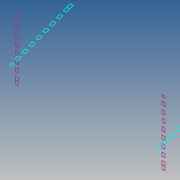
# Autodesk Inventor part: KB33-046-004-017 - Крышка наклонная
Saved by Autodesk Inventor 2020 (Build 240168000, 168)
## iProperties
Created: 2021-06-26
Part Number: KB33-046-004-017 - Крышка наклонная
Material: Типовые
Document SubType Name: Modeling
Designer: Петров Иван
Mass: 69.7839 g
Surface Area: 377.297 cm^2
Volume: 69.7839 cm^3
Density: 1 g/cm^3
Appearance: По умолчанию
Author: Петров Иван
Autodesk Inventor part; units mm, degrees
ref_plane "YZ Plane" through (0, 0, 0) normal (1, 0, 0) x (0, 1, 0)
ref_plane "XZ Plane" through (0, 0, 0) normal (0, 1, 0) x (-1, 0, 0)
ref_plane "XY Plane" through (0, 0, 0) normal (0, 0, 1) x (1, 0, 0)
sketch "Эскиз1" plane through (0, 0, 0) normal (0, 0, 1) x (1, 0, 0)
  line L0 (0, -87.7141) -> (4, -87.7141) projected
  line L1 (4, -87.7141) -> (4, -82.7141) projected
  line L2 (4, -82.7141) -> (0, -82.7141) projected
  line L3 (0, -82.7141) -> (0, -87.7141) projected
  line L4 (4, -77.7141) -> (0, -77.7141) projected
  line L5 (0, -82.7141) -> (0, -77.7141) projected
  line L6 (0, -82.7141) -> (4, -82.7141) projected
  line L7 (4, -77.7141) -> (4, -82.7141) projected
  line L8 (4, -67.7141) -> (0, -67.7141) projected
  line L9 (0, -72.7141) -> (0, -67.7141) projected
  line L10 (0, -72.7141) -> (4, -72.7141) projected
  line L11 (4, -67.7141) -> (4, -72.7141) projected
  line L12 (4, -57.7141) -> (0, -57.7141) projected
  line L13 (0, -62.7141) -> (0, -57.7141) projected
  line L14 (0, -62.7141) -> (4, -62.7141) projected
  line L15 (4, -57.7141) -> (4, -62.7141) projected
  line L16 (4, -47.7141) -> (0, -47.7141) projected
  line L17 (0, -52.7141) -> (0, -47.7141) projected
  line L18 (0, -52.7141) -> (4, -52.7141) projected
  line L19 (4, -47.7141) -> (4, -52.7141) projected
  line L20 (4, -37.7141) -> (0, -37.7141) projected
  line L21 (0, -42.7141) -> (0, -37.7141) projected
  line L22 (0, -42.7141) -> (4, -42.7141) projected
  line L23 (4, -37.7141) -> (4, -42.7141) projected
  line L24 (4, -27.7141) -> (0, -27.7141) projected
  line L25 (0, -32.7141) -> (0, -27.7141) projected
  line L26 (0, -32.7141) -> (4, -32.7141) projected
  line L27 (4, -27.7141) -> (4, -32.7141) projected
  line L28 (4, -17.7141) -> (0, -17.7141) projected
  line L29 (0, -22.7141) -> (0, -17.7141) projected
  line L30 (0, -22.7141) -> (4, -22.7141) projected
  line L31 (4, -17.7141) -> (4, -22.7141) projected
  line L32 (4, -7.7141) -> (0, -7.7141) projected
  line L33 (0, -12.7141) -> (0, -7.7141) projected
  line L34 (0, -12.7141) -> (4, -12.7141) projected
  line L35 (4, -7.7141) -> (4, -12.7141) projected
  line L36 (0, -2.7141) -> (4, -2.7141) projected
  line L37 (4, 0) -> (4, -2.7141) projected
  line L38 (0, 0) -> (4, 0) projected
  line L39 (0, -2.7141) -> (0, 0) projected
  line L40 (-199, -2.7141) -> (-195, -2.7141) projected
  line L41 (-195, 0) -> (-195, -2.7141) projected
  line L42 (-199, 0) -> (-195, 0) projected
  line L43 (-199, -2.7141) -> (-199, 0) projected
  line L44 (-195, -7.7141) -> (-199, -7.7141) projected
  line L45 (-199, -12.7141) -> (-199, -7.7141) projected
  line L46 (-199, -12.7141) -> (-195, -12.7141) projected
  line L47 (-195, -7.7141) -> (-195, -12.7141) projected
  line L48 (-195, -17.7141) -> (-199, -17.7141) projected
  line L49 (-199, -22.7141) -> (-199, -17.7141) projected
  line L50 (-199, -22.7141) -> (-195, -22.7141) projected
  line L51 (-195, -17.7141) -> (-195, -22.7141) projected
  line L52 (-195, -27.7141) -> (-199, -27.7141) projected
  line L53 (-199, -32.7141) -> (-199, -27.7141) projected
  line L54 (-199, -32.7141) -> (-195, -32.7141) projected
  line L55 (-195, -27.7141) -> (-195, -32.7141) projected
  line L56 (-195, -77.7141) -> (-199, -77.7141) projected
  line L57 (-199, -82.7141) -> (-199, -77.7141) projected
  line L58 (-199, -82.7141) -> (-195, -82.7141) projected
  line L59 (-195, -77.7141) -> (-195, -82.7141) projected
  line L60 (-195, -67.7141) -> (-199, -67.7141) projected
  line L61 (-199, -72.7141) -> (-199, -67.7141) projected
  line L62 (-199, -72.7141) -> (-195, -72.7141) projected
  line L63 (-195, -67.7141) -> (-195, -72.7141) projected
  line L64 (-195, -57.7141) -> (-199, -57.7141) projected
  line L65 (-199, -62.7141) -> (-199, -57.7141) projected
  line L66 (-199, -62.7141) -> (-195, -62.7141) projected
  line L67 (-195, -57.7141) -> (-195, -62.7141) projected
  line L68 (-199, -52.7141) -> (-199, -47.7141) projected
  line L69 (-195, -47.7141) -> (-199, -47.7141) projected
  line L70 (-199, -52.7141) -> (-199, -47.7141) projected
  line L71 (-199, -52.7141) -> (-195, -52.7141) projected
  line L72 (-195, -47.7141) -> (-195, -52.7141) projected
  line L73 (-195, -37.7141) -> (-199, -37.7141) projected
  line L74 (-199, -42.7141) -> (-199, -37.7141) projected
  line L75 (-199, -42.7141) -> (-195, -42.7141) projected
  line L76 (-195, -37.7141) -> (-195, -42.7141) projected
  line L77 (-195, -82.7141) -> (-199, -82.7141) projected
  line L78 (-199, -82.7141) -> (-199, -87.7141) projected
  line L79 (-199, -87.7141) -> (-195, -87.7141) projected
  line L80 (-195, -87.7141) -> (-195, -82.7141) projected
  line L81 (-195, 0) -> (0, 0)
  line L82 (0, 0) -> (0, -87.7141)
  line L83 (0, -87.7141) -> (-195, -87.7141)
  line L84 (-195, -87.7141) -> (-195, 0)
  constraints: 8 end point, 2 parallel, 1 horizontal, 1 perpendicular
extrude "Выдавливание1" add sketch "Эскиз1" along normal blind 4 contours L83 L80 L59 L84 L63 L67 L72 L76 L55 L51 L47 L41 L81 L39 L82 L33 L29 L25 L21 L17 L13 L9 L5 L3 | L5 L4 L7 L2 | L58 L57 L56 L59 | L9 L8 L11 L10 | L62 L61 L60 L63 | L13 L12 L15 L14 | L66 L65 L64 L67 | L17 L16 L19 L18 | L71 L68 L69 L72 | L21 L20 L23 L22 | L75 L74 L73 L76 | L25 L24 L27 L26 | L54 L53 L52 L55 | L29 L28 L31 L30 | L50 L49 L48 L51 | L33 L32 L35 L34 | L46 L45 L44 L47 | L39 L38 L37 L36 | L40 L43 L42 L41
